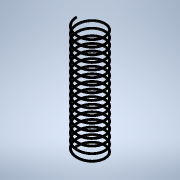
# Autodesk Inventor part: Resorte
Saved by Autodesk Inventor 2020.2 (Build 242310000, 310)
## iProperties
Created: 2019-09-21
Part Number: Resorte
Material: Genérico
Document SubType Name: Modeling
Designer: axelj
Density: 1 g/cm^3
Appearance: Anodizado - Negro
Author: axelj
Autodesk Inventor part; units mm, degrees
ref_plane "YZ Plane" through (0, 0, 0) normal (1, 0, 0) x (0, 1, 0)
ref_plane "XZ Plane" through (0, 0, 0) normal (0, 1, 0) x (-1, 0, 0)
ref_plane "XY Plane" through (0, 0, 0) normal (0, 0, 1) x (1, 0, 0)
sketch "Boceto4" plane through (0, 0, 0) normal (0, 0, 1) x (1, 0, 0)
  line L0 (-6.8981, 0) -> (-7.9869, 0)
  circle A0 centre (-7.4425, 0) radius 0.5444
  point P0 (0, 0)
  constraints: 2 end point, 1 horizontal, 1 horizontal alignment, 1 midpoint, 2 other
sketch "Boceto3" plane through (0, 0, 0) normal (1, 0, 0) x (0, 1, 0)
  line L0 (0, 0) -> (-60.8, 0)
  line L1 (0, 0) -> (20, 0)
  dimension "d1" = 60.8
  dimension "d3" = 20
  constraints: 4 end point, 2 horizontal
  measures "d1" distance of L0.start L0.end
  measures "d3" distance of L0.start L1.end
coil "Bobina1" sketch "Boceto4" operation add axis through (0, 0, 0) along (0, -1, 0) pitch 3.5294 turns 17 hand left
